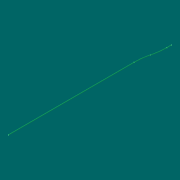
# Autodesk Inventor part: Fiber Loop
Saved by Autodesk Inventor 2016 SP1 (Build 200210100, 210)
## iProperties
Created: 2015-08-17
Part Number: Fiber Loop
Material: Glass
Document SubType Name: Modeling
Designer: Cosmic
Density: 2.18 g/cm^3
Appearance: Clear - Green 1
Author: Cosmic
Autodesk Inventor part; units mm, degrees
ref_plane "YZ Plane" through (0, 0, 0) normal (1, 0, 0) x (0, 1, 0)
ref_plane "XZ Plane" through (0, 0, 0) normal (0, 1, 0) x (-1, 0, 0)
ref_plane "XY Plane" through (0, 0, 0) normal (0, 0, 1) x (1, 0, 0)
sketch "Sketch3" plane through (0, 0, 0) normal (1, 0, 0) x (0, 1, 0)
  line L0 (0, 0) -> (151.8445, 0)
  arc A0 (171.6222, -2.2) -> (151.8445, 0) centre (151.8445, -90) ccw
  arc A1 (171.6222, -2.2) -> (191.4, -4.4) centre (191.4, 85.6) ccw
  line L1 (191.4, -4.4) -> (197, -4.4)
  line L2 (0, 1) -> (151.8445, 1)
  arc A2 (171.842, -1.2244) -> (151.8445, 1) centre (151.8445, -90) ccw
  arc A3 (171.842, -1.2244) -> (191.4, -3.4) centre (191.4, 85.6) ccw
  line L3 (191.4, -3.4) -> (197, -3.4)
  line L4 (197, -4.4) -> (197, -3.4)
  line L5 (0, 0) -> (0, 1)
  dimension "d42" = 90
  dimension "d43" = 90
  dimension "d44" = 4.4
  dimension "d45" = 5.6
  dimension "d46" = 1
  dimension "d50" = 197
  constraints: 12 end point, 8 point on circle, 4 centre point, 3 tangent, 2 horizontal, 1 coincident, 1 parallel, 1 vertical, 3 other
  measures "d42" radius of A0
  measures "d43" radius of A1
  measures "d44" distance between parallel lines of L0 L1
  measures "d45" distance of L1.start L1.end
  measures "d46" distance between parallel lines of L1 L3
  measures "d50" distance between parallel lines of L5 L4
extrude "Extrusion3" add sketch "Sketch3" along normal blind 1
fillet "Fillet2" radius 0.5 16 edges at (1, 181.5607, -2.8544) (1, 161.9049, 0.4422) (1, 75.9222, 1) (1, 194.2, -3.4) (0, 181.5607, -2.8544) (0, 161.9049, 0.4422) (0, 75.9222, 1) (0, 194.2, -3.4) (0, 181.4501, -3.8483) (0, 161.7943, -0.5517) (0, 75.9222, 0) (0, 194.2, -4.4) (1, 181.4501, -3.8483) (1, 161.7943, -0.5517) (1, 75.9222, 0) (1, 194.2, -4.4)
equation "\"d42\" = LoopSmallTrackDiameter"
equation "\"d43\" = LoopSmallTrackDiameter"
equation "\"d44\" = DeepTrackDepth - ShallowTrackDepth"
equation "\"d45\" = DeepTrackDepth"
equation "\"d46\" = OpticalFiberDiameter"
equation "\"d50\" = ScintillatorHeight - ScintillatorEdgeClearence"
equation "\"d47\" = OpticalFiberDiameter"
equation "\"d49\" = 0.5 * OpticalFiberDiameter"
equation "\"OpticalFiberDiameter\" = 1"
equation "\"OpticalFiberClearence\" = 0.1"
equation "\"ScintillatorEdgeClearence\" = 3"
equation "\"MPPCDepth\" = 1"
equation "\"LoopLargeTrackRatio\" = 1.1"
equation "\"LoopSmallTrackDiameter\" = 90"
equation "\"d24\" = 0.05"
equation "\"d25\" = 1"
equation "\"d32\" = 0.05"
equation "\"d33\" = 1"
equation "\"FiberSensorClerence\" = 0.5"
equation "\"SmallTrackDiameter\" = 175"
equation "\"ScintillatorWidth\" = 25"
equation "\"ScintillatorHeight\" = 200"
equation "\"ShallowTrackDepth\" = 1.2"
equation "\"MPPCClearence\" = 0.075"
equation "\"MPPCSensorClearence\" = 1.45"
equation "\"MPPCSensorOffsett\" = 2.105"
equation "\"MPPCWidth\" = 5.9"
equation "\"MPPCHeight\" = 6.55"
equation "\"FiberEdgeOffsett\" = 5"
equation "\"LongFiberAngle\" = 30deg"
equation "\"ShortFiberAngle\" = 78deg"
equation "\"MountingScrewOffsett\" = 9"
equation "\"MountingScrewDepth\" = 4"
equation "\"DeepTrackDepth\" = 5.6"
equation "\"FoilThickness\" = 0.2"
equation "\"silveringThickness\" = 0.2"
equation "\"rubberizedCoating\" = 0.5"
body "Solid2"
